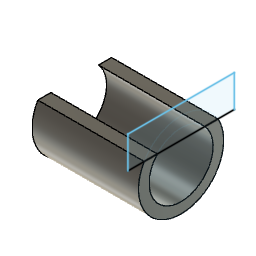
attache_supplémentaire_tige (Autodesk Fusion 360 design; units mm, degrees)
Autodesk Fusion 360 part; units mm, degrees
sketch "Esquisse1" plane through (0, 0, 0) normal (1, 0, 0) x (0, 1, 0)
  circle A0 centre (0, 0) radius 1.5
  circle A1 centre (0, 0) radius 2
  dimension "d1" = 3
  dimension "d2" = 4
  constraint coincident A0.centre A1.centre
  measures "d1" diameter of A0
  measures "d2" diameter of A1
extrude "Extrusion1" add sketch "Esquisse1" along normal blind 5
sketch "Esquisse2" plane through (5, 0, 0) normal (1, 0, 0) x (0, 1, 0)
  circle A0 centre (0, 0) radius 1.5
  circle A1 centre (0, 0) radius 2
  line L0 (-2.5, 2.5) -> (2.5, 2.5)
  line L1 (2.5, 2.5) -> (2.5, 1)
  line L2 (2.5, 1) -> (-2.5, 1)
  line L3 (-2.5, 1) -> (-2.5, 2.5)
  dimension "d5" = 1
  constraint horizontal L0
  constraint vertical L1
  constraint horizontal L2
  constraint vertical L3
  measures "d5" distance of A0.centre L2
extrude "Extrusion2" cut sketch "Esquisse2" against normal blind 15.5 contours A0 L2 | A0 A1 L2 | A1 L0 L1 L2 L3 picked at (0.0881, 1.1959) picked at (-1.3473, 1.2377)
